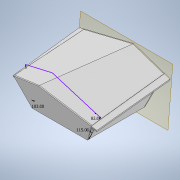
# Autodesk Inventor part: fuckeduphouse
Saved by Autodesk Inventor 2020 (Build 240168000, 168)
## iProperties
Created: 2020-06-23
Part Number: fuckeduphouse
Material: Generic
Document SubType Name: Modeling
Designer: Kitte_x
Density: 1 g/cm^3
Appearance: Default
Author: Kitte_x
Autodesk Inventor part; units mm, degrees
ref_plane "YZ Plane" through (0, 0, 0) normal (1, 0, 0) x (0, 1, 0)
sketch "Sketch1" plane through (0, 0, 0) normal (0, 0, 1) x (1, 0, 0)
  line L0 (-390, -316.4133) -> (390, -316.4133)
  line L1 (390, -316.4133) -> (624.3014, 186.0477)
  line L2 (624.3014, 186.0477) -> (178.4515, 322.3577)
  line L3 (178.4515, 322.3577) -> (-501.2441, 165.4377)
  line L4 (-501.2441, 165.4377) -> (-390, -316.4133)
  point P0 (0, 0)
  point P1 (0, -316.4133)
  dimension "d4" = 780
  dimension "d5" = 103
  dimension "d6" = 150
  dimension "d7" = 82
  dimension "d8" = 115
  dimension "d9" = 90
  constraints: 10 end point, 1 horizontal, 1 midpoint, 1 perpendicular, 1 vertical alignment
  measures "d4" distance of L0.start L0.end
  measures "d5" angle of L0 L4
  measures "d6" angle of L2 L3
  measures "d7" angle of L2 L1
  measures "d8" angle of L1 L0
  measures "d9" angle of L4 L3
ref_plane "Work Plane1" through (0, 0, 780) normal (0, 0, 1) x (1, 0, 0)
sketch "Sketch2" plane through (0, 0, 780) normal (0, 0, 1) x (1, 0, 0)
  line L0 (-390, -316.4133) -> (390, -316.4133) projected
  line L1 (-390, -316.4133) -> (-498.3914, 153.0812)
  line L2 (-498.3914, 153.0812) -> (-120.8416, 240.2454)
  line L3 (-120.8416, 240.2454) -> (553.4449, 34.0954)
  line L4 (553.4449, 34.0954) -> (390, -316.4133)
  point P0 (0, 0)
  dimension "d14" = 82
  dimension "d57" = 103
  dimension "d58" = 115
  constraints: 8 end point, 1 perpendicular
  measures "d14" angle of L4 L3
  measures "d57" angle of L1 L0
  measures "d58" angle of L0 L4
ref_plane "Work Plane2" through (-390, -316.4133, 0) normal (0, 0.0871557, 0.9961947) x (1, 0, 0)
sketch "Sketch6" plane through (-390, -316.4133, 0) normal (0, 0.0871557, 0.9961947) x (1, 0, 0)
  line L0 (568.4515, 641.2111) -> (1014.3014, 504.3804) projected
  line L1 (-111.2441, 483.6916) -> (568.4515, 641.2111) projected
  line L2 (0, 0) -> (-111.2441, 483.6916) projected
  line L3 (0, 0) -> (780, 0) projected
  line L4 (1014.3014, 504.3804) -> (780, 0) projected
  point P0 (390, 315.2093)
extrude "Extrusion2" add sketch "Sketch6" against normal blind 12.7
ref_plane "Work Plane3" through (-390, -316.4133, 780) normal (0, -0.3420201, 0.9396926) x (1, 0, 0)
sketch "Sketch7" plane through (-390, -316.4133, 780) normal (0, -0.3420201, 0.9396926) x (1, 0, 0)
  line L0 (-108.3914, 441.1806) -> (269.1584, 523.0881) projected
  line L1 (0, 0) -> (-108.3914, 441.1806) projected
  line L2 (269.1584, 523.0881) -> (943.4449, 329.3704) projected
  line L3 (943.4449, 329.3704) -> (780, 0) projected
  line L4 (-108.3914, 441.1806) -> (0, 0)
  line L5 (780, 0) -> (0, 0)
  line L6 (780, 0) -> (943.4449, 329.3704)
  line L7 (943.4449, 329.3704) -> (269.1584, 523.0881)
  line L8 (269.1584, 523.0881) -> (-108.3914, 441.1806)
  point P0 (390, 30.5555)
  constraints: 10 end point, 1 collinear, 1 horizontal
loft "Loft3" add profiles "Sketch7" section 2 edges at (401.3765, 254.2027, -49.9224) (-161.3963, 243.8977, -49.0209) (-445.622, -75.4878, -21.0782) (0, -316.4133, 0) (507.1507, -65.1828, -21.9798)
sketch "Sketch8" plane through (-390, -316.4133, 0) normal (0, 0.0871557, 0.9961947) x (1, 0, 0)
  line L0 (568.4515, 641.2111) -> (1014.3014, 504.3804) construction
  line L1 (1014.3014, 504.3804) -> (780, 0) construction
  line L2 (780, 0) -> (0, 0) construction
  line L3 (0, 0) -> (-111.2441, 483.6916) construction
  line L4 (-111.2441, 483.6916) -> (568.4515, 641.2111) construction
  line L5 (567.991, 628.0678) -> (996.6442, 496.5147)
  line L6 (996.6442, 496.5147) -> (771.8962, 12.7)
  line L7 (771.8962, 12.7) -> (10.1107, 12.7)
  line L8 (10.1107, 12.7) -> (-96.0254, 474.1819)
  line L9 (-96.0254, 474.1819) -> (567.991, 628.0678)
  point P0 (390, 315.2093)
  dimension "d37" = 12.7
  constraints: 10 end point, 4 other
  measures "d37" distance between parallel lines of L4 L9
sketch "Sketch9" plane through (-390, -316.4133, 780) normal (0, -0.3420201, 0.9396926) x (1, 0, 0)
  line L0 (-108.3914, 441.1806) -> (0, 0) construction
  line L1 (0, 0) -> (780, 0) construction
  line L2 (780, 0) -> (943.4449, 329.3704) construction
  line L3 (943.4449, 329.3704) -> (269.1584, 523.0881) construction
  line L4 (269.1584, 523.0881) -> (-108.3914, 441.1806) construction
  line L5 (268.7255, 509.9988) -> (925.2973, 321.3704)
  line L6 (925.2973, 321.3704) -> (772.1245, 12.7)
  line L7 (772.1245, 12.7) -> (9.9575, 12.7)
  line L8 (9.9575, 12.7) -> (-92.9442, 431.5363)
  line L9 (-92.9442, 431.5363) -> (268.7255, 509.9988)
  point P0 (390, 30.5555)
  dimension "d38" = 12.7
  constraints: 10 end point, 4 other
  measures "d38" distance between parallel lines of L3 L5
loft "Loft4" cut profiles "Sketch8", "Sketch9"
sketch "Sketch10" plane through (-390, -316.4133, 780) normal (0, -0.3420201, 0.9396926) x (1, 0, 0)
  line L0 (943.4449, 329.3704) -> (269.1584, 523.0881) projected
  line L1 (269.1584, 523.0881) -> (-108.3914, 441.1806) projected
  line L2 (-108.3914, 441.1806) -> (0, 0) projected
  line L3 (0, 0) -> (780, 0) projected
  line L4 (780, 0) -> (943.4449, 329.3704) projected
  point P0 (390, 30.5555)
extrude "Extrusion3" add sketch "Sketch10" along normal blind 12.7
sketch "Sketch11" plane through (-390, -317.5202, -12.6517) normal (0, -0.0871557, -0.9961947) x (-1, 0, 0)
  line L0 (-1014.3014, 504.3804) -> (-568.4515, 641.2111) projected
  line L1 (-1014.3014, 504.3804) -> (-1094.5, 479.7676)
  line L2 (-1094.5, 479.7676) -> (-1087.0478, 455.4854)
  line L3 (-1087.0478, 455.4854) -> (-1003.4992, 481.1263)
  line L4 (-780, 0) -> (-1014.3014, 504.3804) projected
  line L5 (-943.4449, 230.5295) -> (-1014.3014, 504.3804) projected
  line L6 (-1003.4992, 481.1263) -> (-1014.3014, 504.3804)
  point P0 (-390, 315.2093)
  dimension "d46" = 25.4
  constraints: 8 end point, 2 perpendicular, 1 collinear, 1 point on line
  measures "d46" distance between parallel lines of L3 L1
sketch "Sketch12" plane through (-390, -320.757, 791.9341) normal (0, -0.3420201, 0.9396926) x (1, 0, 0)
  line L0 (943.4449, 329.3704) -> (1014.3014, 190.3481) projected
  line L1 (943.4449, 329.3704) -> (1015.1476, 308.7708)
  line L2 (943.4449, 329.3704) -> (269.1584, 523.0881) projected
  line L3 (1015.1476, 308.7708) -> (1008.134, 284.3583)
  line L4 (1008.134, 284.3583) -> (931.967, 306.2405)
  line L5 (780, 0) -> (943.4449, 329.3704) projected
  line L6 (931.967, 306.2405) -> (943.4449, 329.3704)
  point P0 (390, 30.5555)
  dimension "d45" = 25.4
  constraints: 8 end point, 2 collinear, 2 perpendicular, 1 point on line
  measures "d45" distance between parallel lines of L1 L4
loft "Loft5" add profiles "Sketch12", "Sketch11"
sketch "Sketch13" plane through (-390, -320.757, 791.9341) normal (0, -0.3420201, 0.9396926) x (1, 0, 0)
  line L0 (269.1584, 523.0881) -> (-108.3914, 441.1806) projected
  line L1 (-108.3914, 441.1806) -> (-120.6022, 438.5315)
  line L2 (-120.6022, 438.5315) -> (-115.217, 413.7089)
  line L3 (-115.217, 413.7089) -> (-103.0062, 416.358)
  line L4 (-108.3914, 441.1806) -> (0, 0) projected
  line L5 (-103.0062, 416.358) -> (-108.3914, 441.1806)
  point P0 (390, 30.5555)
  dimension "d51" = 25.4
  constraints: 8 end point, 3 perpendicular, 1 collinear
  measures "d51" distance between parallel lines of L1 L3
sketch "Sketch14" plane through (-390, -317.5202, -12.6517) normal (0, -0.0871557, -0.9961947) x (-1, 0, 0)
  line L0 (-568.4515, 641.2111) -> (111.2441, 483.6916) projected
  line L1 (111.2441, 483.6916) -> (180.9234, 467.5434)
  line L2 (180.9234, 467.5434) -> (175.1889, 442.7992)
  line L3 (175.1889, 442.7992) -> (105.5096, 458.9474)
  line L4 (108.3914, 331.8639) -> (111.2441, 483.6916) projected
  line L5 (105.5096, 458.9474) -> (111.2441, 483.6916)
  point P0 (-390, 315.2093)
  dimension "d52" = 25.4
  constraints: 8 end point, 3 perpendicular, 1 collinear
  measures "d52" distance between parallel lines of L3 L1
loft "Loft6" add profiles "Sketch13", "Sketch14"
body "Solid1"
